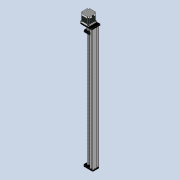
# Autodesk Inventor part: Z Axis Vertical Actuator
Saved by Autodesk Inventor 2022 (Build 260153000, 153)
## iProperties
Created: 2021-10-24
Part Number: Z Axis Vertical Actuator
Material: Generic
Document SubType Name: Modeling
Designer: Coy
Density: 1 g/cm^3
Appearance: Chrome - Polished
Author: Coy
Autodesk Inventor part; units mm, degrees
ref_plane "YZ Plane" through (0, 0, 0) normal (1, 0, 0) x (0, 1, 0)
ref_plane "XZ Plane" through (0, 0, 0) normal (0, 1, 0) x (-1, 0, 0)
ref_plane "XY Plane" through (0, 0, 0) normal (0, 0, 1) x (1, 0, 0)
sketch "Sketch1" plane through (0, 0, 0) normal (0, 1, 0) x (-1, 0, 0)
  line L0 (0, 0) -> (65, 0)
  line L1 (65, 0) -> (65, 42)
  line L2 (65, 42) -> (0, 42)
  line L3 (0, 42) -> (0, 0)
  dimension "d0" = 65
  dimension "d1" = 42
  constraints: 8 end point, 2 parallel, 1 horizontal, 1 perpendicular
  measures "d0" distance of L2.end L1.end
  measures "d1" distance of L1.end L0.end
extrude "Extrusion1" add sketch "Sketch1" along normal blind 9
fillet "Fillet1" radius 5 2 edges at (-65, 4.5, 42) (-65, 4.5, 0)
sketch "Sketch2" plane through (0, 9, 0) normal (0, 1, 0) x (1, 0, 0)
  line L0 (-20, -26.1998) -> (-18.2, -27.9998)
  line L1 (-18.2, -27.9998) -> (-18.2, -25.7897)
  line L2 (-18.2, -25.7897) -> (-16.2, -25.7897)
  line L3 (-16.2, -25.7897) -> (-14, -27.9897)
  line L4 (-14, -27.9897) -> (-14, -30.4998)
  line L5 (-13.5, -30.9998) -> (-14, -30.4998)
  line L6 (-14, -31.4998) -> (-13.5, -30.9998)
  line L7 (-14, -31.4998) -> (-14, -34.0098)
  line L8 (-14, -34.0098) -> (-16.2, -36.2098)
  line L9 (-16.2, -36.2098) -> (-18.2, -36.2098)
  line L10 (-18.2, -36.2098) -> (-18.2, -33.9998)
  line L11 (-18.2, -33.9998) -> (-20, -35.7998)
  line L12 (-20, -35.7998) -> (-20, -40.9998)
  line L13 (-20, -40.9998) -> (-14.8, -40.9998)
  line L14 (-14.8, -40.9998) -> (-13, -39.1998)
  line L15 (-13, -39.1998) -> (-15.2101, -39.1998)
  line L16 (-15.2101, -39.1998) -> (-15.2101, -37.1998)
  line L17 (-15.2101, -37.1998) -> (-13.0101, -34.9998)
  line L18 (-13.0101, -34.9998) -> (-10.5, -34.9998)
  line L19 (-10, -34.4998) -> (-10.5, -34.9998)
  line L20 (-9.5, -34.9998) -> (-10, -34.4998)
  line L21 (-9.5, -34.9998) -> (-6.99, -34.9998)
  line L22 (-6.99, -34.9998) -> (-4.79, -37.1998)
  line L23 (-4.79, -37.1998) -> (-4.79, -39.1998)
  line L24 (-4.79, -39.1998) -> (-7, -39.1998)
  line L25 (-7, -39.1998) -> (-5.2, -40.9998)
  line L26 (-5.2, -40.9998) -> (0, -40.9998)
  line L27 (0, -40.9998) -> (0, -35.7998)
  line L28 (0, -35.7998) -> (-1.8, -33.9998)
  line L29 (-1.8, -33.9998) -> (-1.8, -36.2098)
  line L30 (-1.8, -36.2098) -> (-3.8, -36.2098)
  line L31 (-3.8, -36.2098) -> (-6, -34.0098)
  line L32 (-6, -34.0098) -> (-6, -31.4998)
  line L33 (-6.5, -30.9998) -> (-6, -31.4998)
  line L34 (-6, -30.4998) -> (-6.5, -30.9998)
  line L35 (-6, -30.4998) -> (-6, -27.9897)
  line L36 (-6, -27.9897) -> (-3.8, -25.7897)
  line L37 (-3.8, -25.7897) -> (-1.8, -25.7897)
  line L38 (-1.8, -25.7897) -> (-1.8, -27.9998)
  line L39 (-1.8, -27.9998) -> (0, -26.1998)
  line L40 (0, -26.1998) -> (0, -15.8826)
  arc A0 (0, -15.8826) -> (-0.0586, -15.7412) centre (-0.2, -15.8826) ccw
  line L41 (-0.0586, -15.7412) -> (-1.4586, -14.3412)
  arc A1 (-1.4586, -14.3412) -> (-1.8, -14.4826) centre (-1.6, -14.4826) ccw
  line L42 (-1.8, -14.4826) -> (-1.8, -16.2098)
  line L43 (-1.8, -16.2098) -> (-3.8, -16.2098)
  line L44 (-3.8, -16.2098) -> (-6, -14.0098)
  line L45 (-6, -14.0098) -> (-6, -11.4998)
  line L46 (-6, -11.4998) -> (-6.5, -10.9998)
  line L47 (-6.5, -10.9998) -> (-6, -10.4998)
  line L48 (-6, -10.4998) -> (-6, -7.9897)
  line L49 (-6, -7.9897) -> (-3.8, -5.7897)
  line L50 (-3.8, -5.7897) -> (-1.8, -5.7897)
  line L51 (-1.8, -5.7897) -> (-1.8, -7.5169)
  arc A2 (-1.8, -7.5169) -> (-1.4586, -7.6583) centre (-1.6, -7.5169) ccw
  line L52 (-1.4586, -7.6583) -> (-0.0586, -6.2583)
  arc A3 (-0.0586, -6.2583) -> (0, -6.1169) centre (-0.2, -6.1169) ccw
  line L53 (0, -6.1169) -> (0, -1.1998)
  arc A4 (0, -1.1998) -> (-0.2, -0.9998) centre (-0.2, -1.1998) ccw
  line L54 (-0.2, -0.9998) -> (-5.1172, -0.9998)
  arc A5 (-5.1172, -0.9998) -> (-5.2586, -1.0583) centre (-5.1172, -1.1998) ccw
  line L55 (-5.2586, -1.0583) -> (-6.6586, -2.4583)
  arc A6 (-6.6586, -2.4583) -> (-6.5172, -2.7998) centre (-6.5172, -2.5998) ccw
  line L56 (-6.5172, -2.7998) -> (-4.79, -2.7998)
  line L57 (-4.79, -2.7998) -> (-4.79, -4.7998)
  line L58 (-4.79, -4.7998) -> (-6.99, -6.9998)
  line L59 (-6.99, -6.9998) -> (-9.5, -6.9998)
  line L60 (-9.5, -6.9998) -> (-10, -7.4998)
  line L61 (-10, -7.4998) -> (-10.5, -6.9998)
  line L62 (-10.5, -6.9998) -> (-13.0101, -6.9998)
  line L63 (-13.0101, -6.9998) -> (-15.2101, -4.7998)
  line L64 (-15.2101, -4.7998) -> (-15.2101, -2.7998)
  line L65 (-15.2101, -2.7998) -> (-13.4829, -2.7998)
  arc A7 (-13.4829, -2.7998) -> (-13.3415, -2.4583) centre (-13.4829, -2.5998) ccw
  line L66 (-13.3415, -2.4583) -> (-14.7415, -1.0583)
  arc A8 (-14.7415, -1.0583) -> (-14.8829, -0.9998) centre (-14.8829, -1.1998) ccw
  line L67 (-14.8829, -0.9998) -> (-19.8, -0.9998)
  arc A9 (-19.8, -0.9998) -> (-20, -1.1998) centre (-19.8, -1.1998) ccw
  line L68 (-20, -1.1998) -> (-20, -6.1169)
  arc A10 (-20, -6.1169) -> (-19.9415, -6.2583) centre (-19.8, -6.1169) ccw
  line L69 (-19.9415, -6.2583) -> (-18.5415, -7.6583)
  arc A11 (-18.5415, -7.6583) -> (-18.2, -7.5169) centre (-18.4, -7.5169) ccw
  line L70 (-18.2, -7.5169) -> (-18.2, -5.7897)
  line L71 (-18.2, -5.7897) -> (-16.2, -5.7897)
  line L72 (-16.2, -5.7897) -> (-14, -7.9897)
  line L73 (-14, -7.9897) -> (-14, -10.4998)
  line L74 (-14, -10.4998) -> (-13.5, -10.9998)
  line L75 (-13.5, -10.9998) -> (-14, -11.4998)
  line L76 (-14, -11.4998) -> (-14, -14.0098)
  line L77 (-14, -14.0098) -> (-16.2, -16.2098)
  line L78 (-16.2, -16.2098) -> (-18.2, -16.2098)
  line L79 (-18.2, -16.2098) -> (-18.2, -14.4826)
  arc A12 (-18.2, -14.4826) -> (-18.5415, -14.3412) centre (-18.4, -14.4826) ccw
  line L80 (-18.5415, -14.3412) -> (-19.9415, -15.7412)
  arc A13 (-19.9415, -15.7412) -> (-20, -15.8826) centre (-19.8, -15.8826) ccw
  line L81 (-20, -15.8826) -> (-20, -26.1998)
  circle A14 centre (-10, -10.9998) radius 2.5
  circle A15 centre (-10, -30.9998) radius 2.5
  line L82 (-1.8, -17.1998) -> (-1.8, -24.7998)
  line L83 (-1.8, -24.7998) -> (-4.79, -24.7998)
  line L84 (-4.79, -24.7998) -> (-6.99, -26.9998)
  line L85 (-6.99, -26.9998) -> (-9.5, -26.9998)
  line L86 (-10, -27.4998) -> (-9.5, -26.9998)
  line L87 (-10.5, -26.9998) -> (-10, -27.4998)
  line L88 (-10.5, -26.9998) -> (-13.0101, -26.9998)
  line L89 (-13.0101, -26.9998) -> (-15.2101, -24.7998)
  line L90 (-15.2101, -24.7998) -> (-18.2, -24.7998)
  line L91 (-18.2, -24.7998) -> (-18.2, -17.1998)
  line L92 (-18.2, -17.1998) -> (-15.2101, -17.1998)
  line L93 (-15.2101, -17.1998) -> (-13.0101, -14.9998)
  line L94 (-13.0101, -14.9998) -> (-10.5, -14.9998)
  line L95 (-10.5, -14.9998) -> (-10, -14.4998)
  line L96 (-10, -14.4998) -> (-9.5, -14.9998)
  line L97 (-9.5, -14.9998) -> (-6.99, -14.9998)
  line L98 (-6.99, -14.9998) -> (-4.79, -17.1998)
  line L99 (-4.79, -17.1998) -> (-1.8, -17.1998)
  circle A16 centre (-10, -30.9998) radius 2
  circle A17 centre (-10, -10.9998) radius 2
  line L100 (-20, -25.7897) -> (-26, -25.7897)
  line L101 (-28, -23.7897) -> (-28, -18.0998)
  line L102 (-26, -16.0998) -> (-20, -16.0998)
  line L103 (-20, -16.0998) -> (-20, -25.7897)
  arc A18 (-28, -23.7897) -> (-26, -25.7897) centre (-26, -23.7897) ccw
  arc A19 (-26, -16.0998) -> (-28, -18.0998) centre (-26, -18.0998) ccw
  line L104 (0, 0) -> (-60, 0) construction
  line L105 (-50, 0) -> (-50, -42) construction
  line L106 (-60, -42) -> (0, -42) construction
  circle A20 centre (-50, -21) radius 7.5
  point P0 (-28, -16.0998)
  dimension "d5" = 8
  dimension "d6" = 2
  dimension "d7" = 50
  dimension "d8" = 15
  constraints: 210 end point, 32 point on circle, 21 centre point, 5 point on line, 4 tangent, 2 parallel, 1 equal radius, 1 horizontal, 1 midpoint, 1 perpendicular, 1 vertical
  measures "d5" distance of point (-28, -16.1) L102.end
  measures "d6" radius of A18
  measures "d7" distance from line of L104.start L105
  measures "d8" diameter of A20
extrude "Extrusion2" add sketch "Sketch2" along normal blind 780.5 contours L81 A13 L80 A12 L79 L78 L77 L76 L75 L74 L73 L72 L71 L70 A11 L69 A10 L68 A9 L67 A8 L66 A7 L65 L64 L63 L62 L61 L60 L59 L58 L57 L56 A6 L55 A5 L54 A4 L53 A3 L52 A2 L51 L50 L49 L48 L47 L46 L45 L44 L43 L42 A1 L41 A0 L40 L39 L38 L37 L36 L35 L34 L33 L32 L31 L30 L29 L28 L27 L26 L25 L24 L23 L22 L21 L20 L19 L18 L17 L16 L15 L14 L13 L12 L11 L10 L9 L8 L7 L6 L5 L4 L3 L2 L1 L0 | L100 A18 L101 A19 L102 L81 | A14 | A15 | A20
thread "Thread1" size "M200x8" class "6g" standard "ANSI Metric M Profile" full length
sketch "Sketch3" plane through (0, 789.5, 0) normal (0, 1, 0) x (1, 0, 0)
  line L0 (-26, -25.7897) -> (-20, -25.7897) projected
  line L1 (-20, -25.7897) -> (-20, -26.1998) projected
  line L2 (-20, -26.1998) -> (-18.2, -27.9998) projected
  line L3 (-18.2, -27.9998) -> (-18.2, -25.7897) projected
  line L4 (-18.2, -25.7897) -> (-16.2, -25.7897) projected
  line L5 (-16.2, -25.7897) -> (-14, -27.9897) projected
  line L6 (-14, -27.9897) -> (-14, -30.4998) projected
  line L7 (-14, -30.4998) -> (-13.5, -30.9998) projected
  line L8 (-13.5, -30.9998) -> (-14, -31.4998) projected
  line L9 (-14, -31.4998) -> (-14, -34.0098) projected
  line L10 (-14, -34.0098) -> (-16.2, -36.2098) projected
  line L11 (-16.2, -36.2098) -> (-18.2, -36.2098) projected
  line L12 (-18.2, -36.2098) -> (-18.2, -33.9998) projected
  line L13 (-18.2, -33.9998) -> (-20, -35.7998) projected
  line L14 (-20, -35.7998) -> (-20, -40.9998) projected
  line L15 (-20, -40.9998) -> (-14.8, -40.9998) projected
  line L16 (-14.8, -40.9998) -> (-13, -39.1998) projected
  line L17 (-13, -39.1998) -> (-15.2101, -39.1998) projected
  line L18 (-15.2101, -39.1998) -> (-15.2101, -37.1998) projected
  line L19 (-15.2101, -37.1998) -> (-13.0101, -34.9998) projected
  line L20 (-13.0101, -34.9998) -> (-10.5, -34.9998) projected
  line L21 (-10.5, -34.9998) -> (-10, -34.4998) projected
  line L22 (-10, -34.4998) -> (-9.5, -34.9998) projected
  line L23 (-9.5, -34.9998) -> (-6.99, -34.9998) projected
  line L24 (-6.99, -34.9998) -> (-4.79, -37.1998) projected
  line L25 (-4.79, -37.1998) -> (-4.79, -39.1998) projected
  line L26 (-4.79, -39.1998) -> (-7, -39.1998) projected
  line L27 (-7, -39.1998) -> (-5.2, -40.9998) projected
  line L28 (-5.2, -40.9998) -> (0, -40.9998) projected
  line L29 (0, -40.9998) -> (0, -35.7998) projected
  line L30 (0, -35.7998) -> (-1.8, -33.9998) projected
  line L31 (-1.8, -33.9998) -> (-1.8, -36.2098) projected
  line L32 (-1.8, -36.2098) -> (-3.8, -36.2098) projected
  line L33 (-3.8, -36.2098) -> (-6, -34.0098) projected
  line L34 (-6, -34.0098) -> (-6, -31.4998) projected
  line L35 (-6, -31.4998) -> (-6.5, -30.9998) projected
  line L36 (-6.5, -30.9998) -> (-6, -30.4998) projected
  line L37 (-6, -30.4998) -> (-6, -27.9897) projected
  line L38 (-6, -27.9897) -> (-3.8, -25.7897) projected
  line L39 (-3.8, -25.7897) -> (-1.8, -25.7897) projected
  line L40 (-1.8, -25.7897) -> (-1.8, -27.9998) projected
  line L41 (-1.8, -27.9998) -> (0, -26.1998) projected
  line L42 (0, -26.1998) -> (0, -15.8826) projected
  arc A0 (0, -15.8826) -> (-0.0586, -15.7412) centre (-0.2, -15.8826) ccw projected
  line L43 (-0.0586, -15.7412) -> (-1.4586, -14.3412) projected
  arc A1 (-1.4586, -14.3412) -> (-1.8, -14.4826) centre (-1.6, -14.4826) ccw projected
  line L44 (-1.8, -14.4826) -> (-1.8, -16.2098) projected
  line L45 (-1.8, -16.2098) -> (-3.8, -16.2098) projected
  line L46 (-3.8, -16.2098) -> (-6, -14.0098) projected
  line L47 (-6, -14.0098) -> (-6, -11.4998) projected
  line L48 (-6, -11.4998) -> (-6.5, -10.9998) projected
  line L49 (-6.5, -10.9998) -> (-6, -10.4998) projected
  line L50 (-6, -10.4998) -> (-6, -7.9897) projected
  line L51 (-6, -7.9897) -> (-3.8, -5.7897) projected
  line L52 (-3.8, -5.7897) -> (-1.8, -5.7897) projected
  line L53 (-1.8, -5.7897) -> (-1.8, -7.5169) projected
  arc A2 (-1.8, -7.5169) -> (-1.4586, -7.6583) centre (-1.6, -7.5169) ccw projected
  line L54 (-1.4586, -7.6583) -> (-0.0586, -6.2583) projected
  arc A3 (-0.0586, -6.2583) -> (0, -6.1169) centre (-0.2, -6.1169) ccw projected
  line L55 (0, -6.1169) -> (0, -1.1998) projected
  arc A4 (0, -1.1998) -> (-0.2, -0.9998) centre (-0.2, -1.1998) ccw projected
  line L56 (-0.2, -0.9998) -> (-5.1172, -0.9998) projected
  arc A5 (-5.1172, -0.9998) -> (-5.2586, -1.0583) centre (-5.1172, -1.1998) ccw projected
  line L57 (-5.2586, -1.0583) -> (-6.6586, -2.4583) projected
  arc A6 (-6.6586, -2.4583) -> (-6.5172, -2.7998) centre (-6.5172, -2.5998) ccw projected
  line L58 (-6.5172, -2.7998) -> (-4.79, -2.7998) projected
  line L59 (-4.79, -2.7998) -> (-4.79, -4.7998) projected
  line L60 (-4.79, -4.7998) -> (-6.99, -6.9998) projected
  line L61 (-6.99, -6.9998) -> (-9.5, -6.9998) projected
  line L62 (-9.5, -6.9998) -> (-10, -7.4998) projected
  line L63 (-10, -7.4998) -> (-10.5, -6.9998) projected
  line L64 (-10.5, -6.9998) -> (-13.0101, -6.9998) projected
  line L65 (-13.0101, -6.9998) -> (-15.2101, -4.7998) projected
  line L66 (-15.2101, -4.7998) -> (-15.2101, -2.7998) projected
  line L67 (-15.2101, -2.7998) -> (-13.4829, -2.7998) projected
  arc A7 (-13.4829, -2.7998) -> (-13.3415, -2.4583) centre (-13.4829, -2.5998) ccw projected
  line L68 (-13.3415, -2.4583) -> (-14.7415, -1.0583) projected
  arc A8 (-14.7415, -1.0583) -> (-14.8829, -0.9998) centre (-14.8829, -1.1998) ccw projected
  line L69 (-14.8829, -0.9998) -> (-19.8, -0.9998) projected
  arc A9 (-19.8, -0.9998) -> (-20, -1.1998) centre (-19.8, -1.1998) ccw projected
  line L70 (-20, -1.1998) -> (-20, -6.1169) projected
  arc A10 (-20, -6.1169) -> (-19.9415, -6.2583) centre (-19.8, -6.1169) ccw projected
  line L71 (-19.9415, -6.2583) -> (-18.5415, -7.6583) projected
  arc A11 (-18.5415, -7.6583) -> (-18.2, -7.5169) centre (-18.4, -7.5169) ccw projected
  line L72 (-18.2, -7.5169) -> (-18.2, -5.7897) projected
  line L73 (-18.2, -5.7897) -> (-16.2, -5.7897) projected
  line L74 (-16.2, -5.7897) -> (-14, -7.9897) projected
  line L75 (-14, -7.9897) -> (-14, -10.4998) projected
  line L76 (-14, -10.4998) -> (-13.5, -10.9998) projected
  line L77 (-13.5, -10.9998) -> (-14, -11.4998) projected
  line L78 (-14, -11.4998) -> (-14, -14.0098) projected
  line L79 (-14, -14.0098) -> (-16.2, -16.2098) projected
  line L80 (-16.2, -16.2098) -> (-18.2, -16.2098) projected
  line L81 (-18.2, -16.2098) -> (-18.2, -14.4826) projected
  arc A12 (-18.2, -14.4826) -> (-18.5415, -14.3412) centre (-18.4, -14.4826) ccw projected
  line L82 (-18.5415, -14.3412) -> (-19.9415, -15.7412) projected
  arc A13 (-19.9415, -15.7412) -> (-20, -15.8826) centre (-19.8, -15.8826) ccw projected
  line L83 (-20, -15.8826) -> (-20, -16.0998) projected
  line L84 (-20, -16.0998) -> (-26, -16.0998) projected
  arc A14 (-26, -16.0998) -> (-28, -18.0998) centre (-26, -18.0998) ccw projected
  line L85 (-28, -18.0998) -> (-28, -23.7897) projected
  arc A15 (-28, -23.7897) -> (-26, -25.7897) centre (-26, -23.7897) ccw projected
  line L86 (-10, -27.4998) -> (-10.5, -26.9998) projected
  line L87 (-10.5, -26.9998) -> (-13.0101, -26.9998) projected
  line L88 (-13.0101, -26.9998) -> (-15.2101, -24.7998) projected
  line L89 (-15.2101, -24.7998) -> (-18.2, -24.7998) projected
  line L90 (-18.2, -24.7998) -> (-18.2, -17.1998) projected
  line L91 (-18.2, -17.1998) -> (-15.2101, -17.1998) projected
  line L92 (-15.2101, -17.1998) -> (-13.0101, -14.9998) projected
  line L93 (-13.0101, -14.9998) -> (-10.5, -14.9998) projected
  line L94 (-10.5, -14.9998) -> (-10, -14.4998) projected
  line L95 (-10, -14.4998) -> (-9.5, -14.9998) projected
  line L96 (-9.5, -14.9998) -> (-6.99, -14.9998) projected
  line L97 (-6.99, -14.9998) -> (-4.79, -17.1998) projected
  line L98 (-4.79, -17.1998) -> (-1.8, -17.1998) projected
  line L99 (-1.8, -17.1998) -> (-1.8, -24.7998) projected
  line L100 (-1.8, -24.7998) -> (-4.79, -24.7998) projected
  line L101 (-4.79, -24.7998) -> (-6.99, -26.9998) projected
  line L102 (-6.99, -26.9998) -> (-9.5, -26.9998) projected
  line L103 (-9.5, -26.9998) -> (-10, -27.4998) projected
  circle A16 centre (-10, -10.9998) radius 2 projected
  circle A17 centre (-10, -30.9998) radius 2 projected
  line L104 (-20, -16.0998) -> (-20, -25.7897)
  point P0 (0, 0)
  constraints: 2 end point, 1 vertical
extrude "Extrusion3" add sketch "Sketch3" along normal blind 44.5 contours L104 L83 A13 L82 A12 L81 L80 L79 L78 L77 L76 L75 L74 L73 L72 A11 L71 A10 L70 A9 L69 A8 L68 A7 L67 L66 L65 L64 L63 L62 L61 L60 L59 L58 A6 L57 A5 L56 A4 L55 A3 L54 A2 L53 L52 L51 L50 L49 L48 L47 L46 L45 L44 A1 L43 A0 L42 L41 L40 L39 L38 L37 L36 L35 L34 L33 L32 L31 L30 L29 L28 L27 L26 L25 L24 L23 L22 L21 L20 L19 L18 L17 L16 L15 L14 L13 L12 L11 L10 L9 L8 L7 L6 L5 L4 L3 L2 L1
sketch "Sketch4" plane through (0, 834, 0) normal (0, 1, 0) x (1, 0, 0)
  line L0 (-75, -49.4998) -> (0, -49.4998)
  line L1 (0, -49.4998) -> (0, 7.5002)
  line L2 (0, 7.5002) -> (-75, 7.5002)
  line L3 (-80, 2.5002) -> (-80, -44.4998)
  line L4 (0, -42) -> (0, 0) construction
  line L5 (-20, -40.9998) -> (-14.8, -40.9998) construction
  arc A0 (-80, -44.4998) -> (-75, -49.4998) centre (-75, -44.4998) ccw
  arc A1 (-75, 7.5002) -> (-80, 2.5002) centre (-75, 2.5002) ccw
  circle A2 centre (-50, -21) radius 7.5 projected
  circle A3 centre (-50, -21) radius 8
  point P0 (-80, 7.5002)
  dimension "d15" = 80
  dimension "d16" = 57
  dimension "d17" = 0
  dimension "d18" = 8.5
  dimension "d19" = 5
  dimension "d20" = 16
  constraints: 8 end point, 4 point on circle, 4 tangent, 3 centre point, 2 parallel, 2 point on line, 1 coincident, 1 equal radius, 1 horizontal, 1 perpendicular
  measures "d15" distance of point (-80, 7.5) L1.end
  measures "d16" distance of L1.end L0.end
  measures "d17" distance between parallel lines of L4 L1
  measures "d18" distance between parallel lines of L5 L0
  measures "d19" radius of A0
  measures "d20" diameter of A3
extrude "Extrusion4" add sketch "Sketch4" along normal blind 9 contours A0 L3 A1 L2 L1 L0
sketch "Sketch5" plane through (-20, 9, 16.0998) normal (-1, 0, 0) x (0, 0, 1)
  line L0 (12.4002, 780.5) -> (-2.5998, 780.5) construction
  line L1 (-15.1, 0) -> (-15.1, 825) projected
  line L2 (24.9, 0) -> (24.9, 825) projected
  line L3 (-15.1, 780.5) -> (24.9, 780.5)
  line L4 (24.9, 780.5) -> (24.9, 800.5)
  line L5 (24.9, 800.5) -> (-15.1, 800.5)
  line L6 (-15.1, 800.5) -> (-15.1, 780.5)
  point P0 (-16.0998, -9)
  dimension "d23" = 20
  constraints: 8 end point, 2 parallel, 2 point on line, 1 horizontal, 1 perpendicular
  measures "d23" distance of L4.end L3.end
extrude "Extrusion5" add sketch "Sketch5" along normal blind 9
sketch "Sketch6" plane through (-28, 9, 23.7897) normal (-1, 0, 0) x (0, 0, 1)
  line L0 (-22.7899, 780.5) -> (-22.5899, 780.5) projected
  line L1 (17.2101, 0) -> (17.2101, 825) projected
  line L2 (-22.7899, 780.5) -> (17.2101, 780.5)
  line L3 (17.2101, 780.5) -> (17.2101, 789.5)
  line L4 (17.2101, 789.5) -> (-22.7899, 789.5)
  line L5 (-22.7899, 789.5) -> (-22.7899, 780.5)
  point P0 (-23.7897, -9)
  point P1 (17.2101, 780.5)
  dimension "d26" = 9
  constraints: 8 end point, 2 parallel, 1 horizontal, 1 perpendicular, 1 point on line
  measures "d26" distance between parallel lines of L2 L4
extrude "Extrusion6" add sketch "Sketch6" along normal blind 36
sketch "Sketch7" plane through (0, 834, 0) normal (0, -1, 0) x (1, 0, 0)
  circle A0 centre (-50, 21) radius 8 projected
  circle A1 centre (-50, 21) radius 10
  point P0 (0, 0)
  dimension "d29" = 20
  constraints: 1 centre point, 1 coincident
  measures "d29" diameter of A1
extrude "Extrusion7" add sketch "Sketch7" along normal up to surface (35.5 mm away) contours A0 | A1
fillet "Fillet2" radius 5 2 edges at (-64, 794, 40.9998) (-64, 794, 0.9998)
sketch "Sketch8" plane through (0, 843, 0) normal (0, 1, 0) x (1, 0, 0)
  line L0 (-74.9998, -49.4998) -> (-24.9998, -49.4998)
  line L1 (-21.4998, -45.9998) -> (-21.4998, 4.0002)
  line L2 (-24.9998, 7.5002) -> (-74.9998, 7.5002)
  line L3 (-78.4998, 4.0002) -> (-78.4998, -45.9998)
  line L4 (-75, -49.4998) -> (0, -49.4998) projected
  line L5 (-78.4998, -49.4998) -> (-21.4998, 7.5002) construction
  circle A0 centre (-50, -21) radius 8 construction
  arc A1 (-78.4998, -45.9998) -> (-74.9998, -49.4998) centre (-74.9998, -45.9998) ccw
  arc A2 (-74.9998, 7.5002) -> (-78.4998, 4.0002) centre (-74.9998, 4.0002) ccw
  arc A3 (-21.4998, 4.0002) -> (-24.9998, 7.5002) centre (-24.9998, 4.0002) ccw
  arc A4 (-24.9998, -49.4998) -> (-21.4998, -45.9998) centre (-24.9998, -45.9998) ccw
  line L6 (-21.5098, 4.0002) -> (-21.5098, -45.9998)
  arc A5 (-24.9998, -49.4898) -> (-21.5098, -45.9998) centre (-24.9998, -45.9998) ccw
  line L7 (-24.9998, -49.4898) -> (-74.9998, -49.4898)
  arc A6 (-78.4898, -45.9998) -> (-74.9998, -49.4898) centre (-74.9998, -45.9998) ccw
  line L8 (-78.4898, -45.9998) -> (-78.4898, 4.0002)
  arc A7 (-74.9998, 7.4902) -> (-78.4898, 4.0002) centre (-74.9998, 4.0002) ccw
  line L9 (-74.9998, 7.4902) -> (-24.9998, 7.4902)
  arc A8 (-21.5098, 4.0002) -> (-24.9998, 7.4902) centre (-24.9998, 4.0002) ccw
  point P0 (0, 0)
  point P1 (-21.4998, -49.4998)
  point P2 (-78.4998, 7.5002)
  point P3 (-74.9998, -49.4998)
  dimension "d33" = 57
  dimension "d34" = 57
  dimension "d35" = 0
  dimension "d36" = 3.5
  dimension "d39" = 0.01
  constraints: 18 end point, 16 point on circle, 9 point on line, 8 centre point, 8 tangent, 4 parallel, 3 equal radius, 2 perpendicular, 1 horizontal, 7 other
  measures "d33" distance of point (-78.5, 7.5) L5.end
  measures "d34" distance of L5.end point (-21.5, -49.5)
  measures "d35" distance between parallel lines of L4 L0
  measures "d36" radius of A1
  measures "d39" distance between parallel lines of L1 L6
extrude "Extrusion8" add sketch "Sketch8" along normal blind 5 contours L6 A5 L7 A6 L8 A7 L9 A8
sketch "Sketch9" plane through (0, 848, 0) normal (0, 1, 0) x (1, 0, 0)
  line L0 (-26.4298, -44.5698) -> (-73.5698, -44.5698) construction
  line L1 (-73.5698, -44.5698) -> (-73.5698, 2.5702) construction
  line L2 (-73.5698, 2.5702) -> (-26.4298, 2.5702) construction
  line L3 (-26.4298, 2.5702) -> (-26.4298, -44.5698) construction
  line L4 (-73.5698, -44.5698) -> (-78.4898, -44.5698) construction
  line L5 (-78.4898, 4.0002) -> (-78.4898, -45.9998) construction
  line L6 (-73.5698, -44.5698) -> (-73.5698, -49.4898) construction
  line L7 (-74.9998, -49.4898) -> (-24.9998, -49.4898) construction
  line L8 (-26.4298, 2.5702) -> (-21.5098, 2.5702) construction
  line L9 (-21.5098, -45.9998) -> (-21.5098, 4.0002) construction
  line L10 (-26.4298, 2.5702) -> (-26.4298, 7.4902) construction
  line L11 (-24.9998, 7.4902) -> (-74.9998, 7.4902) construction
  circle A0 centre (-73.5698, -44.5698) radius 2.5 construction
  circle A1 centre (-73.5698, 2.5702) radius 2.5 construction
  circle A2 centre (-26.4298, 2.5702) radius 2.5 construction
  circle A3 centre (-26.4298, -44.5698) radius 2.5 construction
  arc A4 (-69.5698, -44.5698) -> (-73.5698, -40.5698) centre (-73.5698, -44.5698) ccw
  circle A5 centre (-26.4298, -44.5698) radius 4
  circle A6 centre (-26.4298, 2.5702) radius 4
  line L12 (-69.5698, -44.5698) -> (-69.5698, -48.4898)
  line L13 (-73.5698, -40.5698) -> (-77.4898, -40.5698)
  line L14 (-78.4898, 4.0002) -> (-78.4898, -45.9998) construction
  arc A7 (-78.4898, -45.9998) -> (-74.9998, -49.4898) centre (-74.9998, -45.9998) ccw construction
  line L15 (-74.9998, -49.4898) -> (-24.9998, -49.4898) construction
  arc A8 (-24.9998, -49.4898) -> (-21.5098, -45.9998) centre (-24.9998, -45.9998) ccw construction
  line L16 (-21.5098, -45.9998) -> (-21.5098, 4.0002) construction
  arc A9 (-21.5098, 4.0002) -> (-24.9998, 7.4902) centre (-24.9998, 4.0002) ccw construction
  line L17 (-24.9998, 7.4902) -> (-74.9998, 7.4902) construction
  arc A10 (-74.9998, 7.4902) -> (-78.4898, 4.0002) centre (-74.9998, 4.0002) ccw construction
  arc A11 (-78.4898, -39.5698) -> (-77.4898, -40.5698) centre (-77.4898, -39.5698) ccw
  arc A12 (-69.5698, -48.4898) -> (-68.5698, -49.4898) centre (-68.5698, -48.4898) ccw
  line L18 (-78.4898, -39.5698) -> (-78.4898, -20.9998)
  line L19 (-68.5698, -49.4898) -> (-49.9998, -49.4898)
  line L20 (-49.9998, -49.4898) -> (-49.9998, 7.4902) construction
  circle A13 centre (-50, -21) radius 7.5 construction
  line L21 (-31.4302, -49.4898) -> (-50.0002, -49.4898)
  arc A14 (-31.4302, -49.4898) -> (-30.4302, -48.4898) centre (-31.4302, -48.4898) ccw
  line L22 (-30.4302, -44.5698) -> (-30.4302, -48.4898)
  arc A15 (-26.4302, -40.5698) -> (-30.4302, -44.5698) centre (-26.4302, -44.5698) ccw
  line L23 (-26.4302, -40.5698) -> (-22.5102, -40.5698)
  arc A16 (-22.5102, -40.5698) -> (-21.5102, -39.5698) centre (-22.5102, -39.5698) ccw
  line L24 (-21.5102, -39.5698) -> (-21.5102, -20.9998)
  line L25 (-21.5102, -2.4302) -> (-21.5102, -21.0002)
  arc A17 (-21.5102, -2.4302) -> (-22.5102, -1.4302) centre (-22.5102, -2.4302) ccw
  line L26 (-26.4302, -1.4302) -> (-22.5102, -1.4302)
  arc A18 (-30.4302, 2.5698) -> (-26.4302, -1.4302) centre (-26.4302, 2.5698) ccw
  line L27 (-30.4302, 2.5698) -> (-30.4302, 6.4898)
  arc A19 (-30.4302, 6.4898) -> (-31.4302, 7.4898) centre (-31.4302, 6.4898) ccw
  line L28 (-31.4302, 7.4898) -> (-50.0002, 7.4898)
  line L29 (-68.5698, 7.4898) -> (-49.9998, 7.4898)
  arc A20 (-68.5698, 7.4898) -> (-69.5698, 6.4898) centre (-68.5698, 6.4898) ccw
  line L30 (-69.5698, 2.5698) -> (-69.5698, 6.4898)
  arc A21 (-73.5698, -1.4302) -> (-69.5698, 2.5698) centre (-73.5698, 2.5698) ccw
  line L31 (-73.5698, -1.4302) -> (-77.4898, -1.4302)
  arc A22 (-77.4898, -1.4302) -> (-78.4898, -2.4302) centre (-77.4898, -2.4302) ccw
  line L32 (-78.4898, -2.4302) -> (-78.4898, -21.0002)
  point P0 (0, 0)
  dimension "d40" = 47.14
  dimension "d41" = 47.14
  dimension "d42" = 5
  dimension "d43" = 5
  dimension "d44" = 5
  dimension "d45" = 5
  dimension "d47" = 1.5
  dimension "d48" = 1.5
  dimension "d49" = 1.5
  dimension "d50" = 2
  dimension "d51" = 2
  dimension "d54" = 360
  constraints: 50 end point, 24 point on circle, 18 centre point, 8 point on line, 6 perpendicular, 6 tangent, 5 coincident, 4 parallel, 3 midpoint, 2 horizontal, 73 other
  measures "d40" distance of L1.end L2.end
  measures "d41" distance of L0.end L1.end
  measures "d42" diameter of A0
  measures "d43" diameter of A1
  measures "d44" diameter of A2
  measures "d45" diameter of A3
  measures "d47" radial gap between concentric circles of A0 A4
  measures "d48" radial gap between concentric circles of A3 A5
  measures "d49" radial gap between concentric circles of A2 A6
  measures "d50" diameter of A11
  measures "d51" diameter of A12
extrude "Extrusion9" add sketch "Sketch9" along normal blind 6 contours A4 L13 A11 L18 L32 A22 L31 A21 L30 A20 L29 L28 A19 L27 A6 L26 A17 L25 L24 A16 L23 A5 L22 A14 L21 L19 A12 L12
sketch "Sketch10" plane through (0, 854, 0) normal (0, 1, 0) x (1, 0, 0)
  line L0 (-68.5698, -49.4898) -> (-31.4302, -49.4898) projected
  arc A0 (-31.4302, -49.4898) -> (-30.4302, -48.4898) centre (-31.4302, -48.4898) ccw projected
  line L1 (-30.4302, -48.4898) -> (-30.4302, -44.5698) projected
  arc A1 (-26.4302, -40.5698) -> (-30.4302, -44.5698) centre (-26.4302, -44.5698) ccw projected
  line L2 (-26.4302, -40.5698) -> (-22.5102, -40.5698) projected
  arc A2 (-22.5102, -40.5698) -> (-21.5102, -39.5698) centre (-22.5102, -39.5698) ccw projected
  line L3 (-21.5102, -39.5698) -> (-21.5102, -2.4302) projected
  arc A3 (-21.5102, -2.4302) -> (-22.5102, -1.4302) centre (-22.5102, -2.4302) ccw projected
  line L4 (-22.5102, -1.4302) -> (-26.4302, -1.4302) projected
  arc A4 (-30.4302, 2.5698) -> (-26.4302, -1.4302) centre (-26.4302, 2.5698) ccw projected
  line L5 (-30.4302, 2.5698) -> (-30.4302, 6.4898) projected
  arc A5 (-30.4302, 6.4898) -> (-31.4302, 7.4898) centre (-31.4302, 6.4898) ccw projected
  line L6 (-31.4302, 7.4898) -> (-68.5698, 7.4898) projected
  arc A6 (-68.5698, 7.4898) -> (-69.5698, 6.4898) centre (-68.5698, 6.4898) ccw projected
  line L7 (-69.5698, 6.4898) -> (-69.5698, 2.5698) projected
  arc A7 (-73.5698, -1.4302) -> (-69.5698, 2.5698) centre (-73.5698, 2.5698) ccw projected
  line L8 (-73.5698, -1.4302) -> (-77.4898, -1.4302) projected
  arc A8 (-77.4898, -1.4302) -> (-78.4898, -2.4302) centre (-77.4898, -2.4302) ccw projected
  line L9 (-78.4898, -2.4302) -> (-78.4898, -39.5698) projected
  arc A9 (-78.4898, -39.5698) -> (-77.4898, -40.5698) centre (-77.4898, -39.5698) ccw projected
  line L10 (-77.4898, -40.5698) -> (-73.5698, -40.5698) projected
  arc A10 (-69.5698, -44.5698) -> (-73.5698, -40.5698) centre (-73.5698, -44.5698) ccw projected
  line L11 (-69.5698, -44.5698) -> (-69.5698, -48.4898) projected
  arc A11 (-69.5698, -48.4898) -> (-68.5698, -49.4898) centre (-68.5698, -48.4898) ccw projected
  line L12 (-73.5698, -40.5598) -> (-77.4898, -40.5598)
  arc A12 (-78.4798, -39.5698) -> (-77.4898, -40.5598) centre (-77.4898, -39.5698) ccw
  line L13 (-78.4798, -39.5698) -> (-78.4798, -2.4302)
  arc A13 (-77.4898, -1.4402) -> (-78.4798, -2.4302) centre (-77.4898, -2.4302) ccw
  line L14 (-77.4898, -1.4402) -> (-73.5698, -1.4402)
  arc A14 (-73.5698, -1.4402) -> (-69.5598, 2.5698) centre (-73.5698, 2.5698) ccw
  line L15 (-69.5598, 2.5698) -> (-69.5598, 6.4898)
  arc A15 (-68.5698, 7.4798) -> (-69.5598, 6.4898) centre (-68.5698, 6.4898) ccw
  line L16 (-68.5698, 7.4798) -> (-31.4302, 7.4798)
  arc A16 (-30.4402, 6.4898) -> (-31.4302, 7.4798) centre (-31.4302, 6.4898) ccw
  line L17 (-30.4402, 6.4898) -> (-30.4402, 2.5698)
  arc A17 (-30.4402, 2.5698) -> (-26.4302, -1.4402) centre (-26.4302, 2.5698) ccw
  line L18 (-26.4302, -1.4402) -> (-22.5102, -1.4402)
  arc A18 (-21.5202, -2.4302) -> (-22.5102, -1.4402) centre (-22.5102, -2.4302) ccw
  line L19 (-21.5202, -2.4302) -> (-21.5202, -39.5698)
  arc A19 (-22.5102, -40.5598) -> (-21.5202, -39.5698) centre (-22.5102, -39.5698) ccw
  line L20 (-22.5102, -40.5598) -> (-26.4302, -40.5598)
  arc A20 (-26.4302, -40.5598) -> (-30.4402, -44.5698) centre (-26.4302, -44.5698) ccw
  line L21 (-30.4402, -44.5698) -> (-30.4402, -48.4898)
  arc A21 (-31.4302, -49.4798) -> (-30.4402, -48.4898) centre (-31.4302, -48.4898) ccw
  line L22 (-31.4302, -49.4798) -> (-68.5698, -49.4798)
  arc A22 (-69.5598, -48.4898) -> (-68.5698, -49.4798) centre (-68.5698, -48.4898) ccw
  line L23 (-69.5598, -48.4898) -> (-69.5598, -44.5698)
  arc A23 (-69.5598, -44.5698) -> (-73.5698, -40.5598) centre (-73.5698, -44.5698) ccw
  point P0 (0, 0)
  dimension "d58" = 0.01
  constraints: 24 end point, 24 point on circle, 12 centre point, 23 other
  measures "d58" distance between parallel lines of L10 L12
extrude "Extrusion10" add sketch "Sketch10" along normal blind 33 contours L12 A12 L13 A13 L14 A14 L15 A15 L16 A16 L17 A17 L18 A18 L19 A19 L20 A20 L21 A21 L22 A22 L23 A23
sketch "Sketch11" plane through (0, 887, 0) normal (0, 1, 0) x (1, 0, 0)
  line L0 (-68.5698, -49.4798) -> (-31.4302, -49.4798) projected
  arc A0 (-31.4302, -49.4798) -> (-30.4402, -48.4898) centre (-31.4302, -48.4898) ccw projected
  line L1 (-30.4402, -48.4898) -> (-30.4402, -44.5698) projected
  arc A1 (-26.4302, -40.5598) -> (-30.4402, -44.5698) centre (-26.4302, -44.5698) ccw projected
  line L2 (-26.4302, -40.5598) -> (-22.5102, -40.5598) projected
  arc A2 (-22.5102, -40.5598) -> (-21.5202, -39.5698) centre (-22.5102, -39.5698) ccw projected
  line L3 (-21.5202, -39.5698) -> (-21.5202, -2.4302) projected
  arc A3 (-21.5202, -2.4302) -> (-22.5102, -1.4402) centre (-22.5102, -2.4302) ccw projected
  line L4 (-22.5102, -1.4402) -> (-26.4302, -1.4402) projected
  arc A4 (-30.4402, 2.5698) -> (-26.4302, -1.4402) centre (-26.4302, 2.5698) ccw projected
  line L5 (-30.4402, 2.5698) -> (-30.4402, 6.4898) projected
  arc A5 (-30.4402, 6.4898) -> (-31.4302, 7.4798) centre (-31.4302, 6.4898) ccw projected
  line L6 (-31.4302, 7.4798) -> (-68.5698, 7.4798) projected
  arc A6 (-68.5698, 7.4798) -> (-69.5598, 6.4898) centre (-68.5698, 6.4898) ccw projected
  line L7 (-69.5598, 6.4898) -> (-69.5598, 2.5698) projected
  arc A7 (-73.5698, -1.4402) -> (-69.5598, 2.5698) centre (-73.5698, 2.5698) ccw projected
  line L8 (-73.5698, -1.4402) -> (-77.4898, -1.4402) projected
  arc A8 (-77.4898, -1.4402) -> (-78.4798, -2.4302) centre (-77.4898, -2.4302) ccw projected
  line L9 (-78.4798, -2.4302) -> (-78.4798, -39.5698) projected
  arc A9 (-78.4798, -39.5698) -> (-77.4898, -40.5598) centre (-77.4898, -39.5698) ccw projected
  line L10 (-77.4898, -40.5598) -> (-73.5698, -40.5598) projected
  arc A10 (-69.5598, -44.5698) -> (-73.5698, -40.5598) centre (-73.5698, -44.5698) ccw projected
  line L11 (-69.5598, -44.5698) -> (-69.5598, -48.4898) projected
  arc A11 (-69.5598, -48.4898) -> (-68.5698, -49.4798) centre (-68.5698, -48.4898) ccw projected
  line L12 (-73.5698, -40.5698) -> (-77.4898, -40.5698)
  arc A12 (-78.4898, -39.5698) -> (-77.4898, -40.5698) centre (-77.4898, -39.5698) ccw
  line L13 (-78.4898, -39.5698) -> (-78.4898, -2.4302)
  arc A13 (-77.4898, -1.4302) -> (-78.4898, -2.4302) centre (-77.4898, -2.4302) ccw
  line L14 (-77.4898, -1.4302) -> (-73.5698, -1.4302)
  arc A14 (-73.5698, -1.4302) -> (-69.5698, 2.5698) centre (-73.5698, 2.5698) ccw
  line L15 (-69.5698, 2.5698) -> (-69.5698, 6.4898)
  arc A15 (-68.5698, 7.4898) -> (-69.5698, 6.4898) centre (-68.5698, 6.4898) ccw
  line L16 (-68.5698, 7.4898) -> (-31.4302, 7.4898)
  arc A16 (-30.4302, 6.4898) -> (-31.4302, 7.4898) centre (-31.4302, 6.4898) ccw
  line L17 (-30.4302, 6.4898) -> (-30.4302, 2.5698)
  arc A17 (-30.4302, 2.5698) -> (-26.4302, -1.4302) centre (-26.4302, 2.5698) ccw
  line L18 (-26.4302, -1.4302) -> (-22.5102, -1.4302)
  arc A18 (-21.5102, -2.4302) -> (-22.5102, -1.4302) centre (-22.5102, -2.4302) ccw
  line L19 (-21.5102, -2.4302) -> (-21.5102, -39.5698)
  arc A19 (-22.5102, -40.5698) -> (-21.5102, -39.5698) centre (-22.5102, -39.5698) ccw
  line L20 (-22.5102, -40.5698) -> (-26.4302, -40.5698)
  arc A20 (-26.4302, -40.5698) -> (-30.4302, -44.5698) centre (-26.4302, -44.5698) ccw
  line L21 (-30.4302, -44.5698) -> (-30.4302, -48.4898)
  arc A21 (-31.4302, -49.4898) -> (-30.4302, -48.4898) centre (-31.4302, -48.4898) ccw
  line L22 (-31.4302, -49.4898) -> (-68.5698, -49.4898)
  arc A22 (-69.5698, -48.4898) -> (-68.5698, -49.4898) centre (-68.5698, -48.4898) ccw
  line L23 (-69.5698, -48.4898) -> (-69.5698, -44.5698)
  arc A23 (-69.5698, -44.5698) -> (-73.5698, -40.5698) centre (-73.5698, -44.5698) ccw
  point P0 (0, 0)
  dimension "d61" = 0.01
  constraints: 24 end point, 24 point on circle, 12 centre point, 23 other
  measures "d61" radial gap between concentric circles of A10 A23
extrude "Extrusion11" add sketch "Sketch11" along normal blind 11 contours A11 L11 A10 L10 A9 L9 A8 L8 A7 L7 A6 L6 A5 L5 A4 L4 A3 L3 A2 L2 A1 L1 A0 L0 | L12 A12 L13 A13 L14 A14 L15 A15 L16 A16 L17 A17 L18 A18 L19 A19 L20 A20 L21 A21 L22 A22 L23 A23
sketch "Sketch12" plane through (-21.5102, 887, 39.5698) normal (1, 0, 0) x (0, 0, -1)
  line L0 (0, 0) -> (37.1395, 0) construction
  line L1 (37.1395, 0) -> (37.1395, 11) construction
  line L2 (0, 11) -> (37.1395, 11) construction
  line L3 (0, 0) -> (0, 11) construction
  line L4 (37.1395, 11) -> (0, 11) construction
  line L5 (18.5698, 11) -> (18.5698, 0) construction
  line L6 (37.1395, 0) -> (0, 0) construction
  circle A0 centre (18.5698, 5.5) radius 5.5
  point P0 (39.5698, -887)
  constraints: 3 midpoint, 2 end point, 1 vertical alignment, 2 other
extrude "Extrusion12" add sketch "Sketch12" along normal blind 2
sketch "Sketch13" plane through (0, 848, 0) normal (0, 1, 0) x (1, 0, 0)
  circle A0 centre (-50, -21) radius 8 construction
  circle A1 centre (-50, -21) radius 10 construction
  arc A2 (-78.4898, -45.9998) -> (-74.9998, -49.4898) centre (-74.9998, -45.9998) ccw construction
  arc A3 (-69.5698, -44.5698) -> (-73.5698, -40.5698) centre (-73.5698, -44.5698) ccw construction
  circle A4 centre (-73.5698, -44.5698) radius 3
  circle A5 centre (-26.4302, -44.5698) radius 3
  circle A6 centre (-26.4302, 2.5698) radius 3
  circle A7 centre (-73.5698, 2.5698) radius 3
  point P0 (0, 0)
  dimension "d66" = 6
  dimension "d69" = 360
  constraints: 4 centre point, 1 coincident, 9 other
  measures "d66" diameter of A4
extrude "Extrusion13" add sketch "Sketch13" along normal blind 3.5
sketch "Sketch14" plane through (-14.8, 9, 40.9998) normal (0, 0, 1) x (1, 0, 0)
  line L0 (-44.2, 780.5) -> (-44.2, 789.5) projected
  line L1 (-5.2, 780.5) -> (-44.2, 780.5) projected
  line L2 (-5.2, 0) -> (-5.2, 780.5) projected
  line L3 (0, 0) -> (-5.2, 0) projected
  line L4 (0, 0) -> (0, 825) projected
  line L5 (-5.2, 825) -> (0, 825) projected
  line L6 (-5.2, 800.5) -> (-5.2, 825) projected
  line L7 (-5.2, 800.5) -> (-14.2, 800.5) projected
  line L8 (-14.2, 789.5) -> (-14.2, 800.5) projected
  line L9 (-14.2, 789.5) -> (-44.2, 789.5) projected
  line L10 (-5.2, 800.5) -> (-5.2, 825) projected
  line L11 (-5.2, 800.5) -> (-5.2, 780.5)
  line L12 (-3.4, 0) -> (-3.4, 825) projected
  line L13 (-5.21, 800.5) -> (-5.21, 780.5)
  point P0 (14.8, -9)
  point P1 (-5.21, 800.5)
  point P2 (-5.21, 780.5)
  dimension "d73" = 0.01
  constraints: 4 end point, 2 parallel
  measures "d73" distance between parallel lines of L11 L13
extrude "Extrusion14" cut sketch "Sketch14" against normal blind 0.01 contours L13 L7 L11 L1
equation "\"d43\" = d42"
equation "\"d44\" = d42"
equation "\"d45\" = d42"
body "Solid1"
